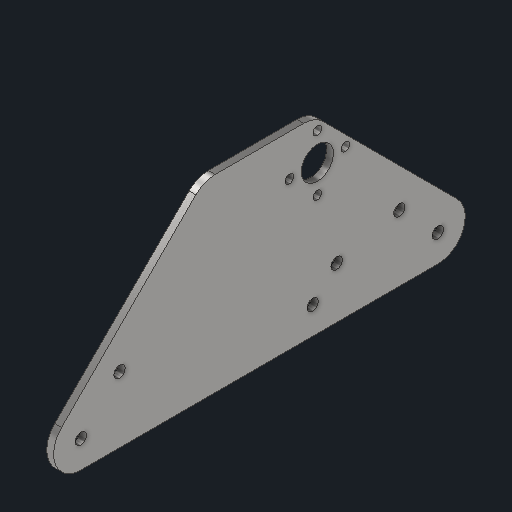
# Autodesk Inventor part: HipPivotPlate
Saved by Autodesk Inventor 2026.1 (Build 301233020, 233B)
## iProperties
Created: 2023-04-06
Part Number: HipPivotPlate
Material: Aluminum 6061
Document SubType Name: Modeling
Designer: Dave
Density: 2.7 g/cm^3
Appearance: Galvanized
Mass: 96.5969 g
Surface Area: 244.776 cm^2
Volume: 35.7766 cm^3
Author: Dave
Autodesk Inventor part; units mm, degrees
ref_plane "YZ Plane" through (0, 0, 0) normal (1, 0, 0) x (0, 1, 0)
ref_plane "XZ Plane" through (0, 0, 0) normal (0, 1, 0) x (-1, 0, 0)
ref_plane "XY Plane" through (0, 0, 0) normal (0, 0, 1) x (1, 0, 0)
sketch "Sketch1" plane through (0, 0, 0) normal (1, 0, 0) x (0, 1, 0)
  circle A0 centre (0, 0) radius 7.5075
  circle A1 centre (-56.0605, -56.0605) radius 2.65
  circle A2 centre (-38.1, -38.1) radius 2.65
  circle A3 centre (-47.0803, 100.9618) radius 2.65
  circle A4 centre (-56.0605, 109.942) radius 2.65
  circle A5 centre (-38.1, 91.9815) radius 2.65
  circle A6 centre (-47.0803, -47.0803) radius 2.65
  line L0 (-47.0803, 100.9618) -> (6.8013, 47.0803) construction
  line L1 (-35.921, 35.921) -> (0, 0) construction
  line L2 (0, 0) -> (-35.921, -35.921) construction
  line L3 (0, 0) -> (12.7, 0) construction
  line L4 (-47.0803, 118.9223) -> (15.3303, 56.5118)
  line L5 (19.05, 47.5315) -> (19.05, 6.35)
  line L6 (-68.7605, -56.0605) -> (-68.7605, 109.942)
  arc A7 (19.05, 47.5315) -> (15.3303, 56.5118) centre (6.35, 47.5315) ccw
  arc A8 (-47.0803, 118.9223) -> (-68.7605, 109.942) centre (-56.0605, 109.942) ccw
  line L7 (-47.0803, -65.0408) -> (15.3303, -2.6303)
  arc A9 (15.3303, -2.6303) -> (19.05, 6.35) centre (6.35, 6.35) ccw
  arc A10 (-68.7605, -56.0605) -> (-47.0803, -65.0408) centre (-56.0605, -56.0605) ccw
  line L8 (-26.9408, -8.9802) -> (-44.9013, -26.9407) projected
  line L9 (-44.9013, -26.9407) -> (-284.0015, 212.1595) projected
  line L10 (-266.041, 230.12) -> (-284.0015, 212.1595) projected
  line L11 (-26.9408, -8.9802) -> (-266.041, 230.12) projected
  circle A11 centre (-56.0605, 2.179) radius 2.65
  circle A12 centre (-44.9013, -8.9802) radius 2.65
  line L12 (-56.0605, 2.179) -> (-44.9013, -8.9802) construction
  point P0 (19.05, 1.0895)
  point P1 (-68.7605, -86.721)
  point P2 (-68.7605, 32.8395)
  dimension "d0" = 15.015
  dimension "d1" = 5.3
  dimension "d2" = 5.3
  dimension "d3" = 5.3
  dimension "d4" = 5.3
  dimension "d5" = 5.3
  dimension "d6" = 5.3
  dimension "d8" = 38.1
  dimension "d10" = 38.1
  dimension "d11" = 12.7
  dimension "d12" = 12.7
  dimension "d13" = 38.1
  dimension "d14" = 12.7
  dimension "d15" = 12.7
  dimension "d16" = 12.7
  dimension "d18" = 19.05
  dimension "d19" = 45
  dimension "d20" = 12.7
  dimension "d21" = 12.7
  dimension "d24" = 12.7
  dimension "d25" = 12.7
  dimension "d27" = 12.7
  dimension "d29" = 12.7
  dimension "d34" = 12.7
  dimension "d47" = 12.7
  dimension "d49" = 50.8
  dimension "d50" = 76.2
  dimension "d51" = 12.7
  constraints: 18 end point, 13 centre point, 9 point on line, 8 point on circle, 8 tangent, 4 parallel, 3 equal radius, 3 perpendicular, 1 coincident, 1 horizontal, 1 vertical
  measures "d0" diameter of A0
  measures "d1" diameter of A1
  measures "d2" diameter of A2
  measures "d3" diameter of A3
  measures "d4" diameter of A4
  measures "d5" diameter of A5
  measures "d6" diameter of A6
  measures "d8" distance between parallel lines of L1 L0
  measures "d10" horizontal distance of A5.centre point (0, 0)
  measures "d11" distance of A5.centre L0.start
  measures "d12" distance of L0.start A4.centre
  measures "d13" horizontal distance of A2.centre point (0, 0)
  measures "d14" distance of A6.centre A2.centre
  measures "d15" distance of A1.centre A6.centre
  measures "d16" distance from line of L4 A5.centre
  measures "d18" distance from line of L5 point (0, 0)
  measures "d19" angle of L5 L4
  measures "d20" distance from line of L6 A4.centre
  measures "d21" radius of A7
  measures "d24" radius of A9
  measures "d25" distance from line of L7 A1.centre
  measures "d27" distance between parallel lines of L11 L12
  measures "d29" distance from line of L8 L12.end
  measures "d34" distance from line of L6 L12.start
  measures "d47" radius of A8
  measures "d49" distance of L1.start L1.end
  measures "d50" distance of L0.start L0.end
  measures "d51" distance of L1.end L3.end
extrude "Extrusion2" add sketch "Sketch1" along normal blind 3.175 contours A3 | A6 | L4 A7 L5 A9 L7 A10 L6 L9 L8 L11 A8 | L11 L8 L9 L6
sketch "Sketch3" plane through (3.175, 0, 0) normal (1, 0, 0) x (0, 0, -1)
  circle A0 centre (0, 0) radius 7.5075 projected
  circle A1 centre (0, 0) radius 13 construction
  circle A2 centre (-0.0008, 13) radius 2
  line L0 (-6.35, 19.05) -> (-47.5315, 19.05) projected
  circle A3 centre (-13, -0.0008) radius 2
  circle A4 centre (0.0008, -13) radius 2
  circle A5 centre (13, 0.0008) radius 2
  dimension "d37" = 26
  dimension "d38" = 4
  dimension "d42" = 360
  constraints: 4 centre point, 3 coincident, 14 other
  measures "d38" diameter of A2
extrude "Extrusion3" cut sketch "Sketch3" against normal blind 25.4 contours A2 | A3 | A4 | A5
equation "\"d12\" = d11"
equation "\"d13\" = d10"
equation "\"d14\" = d11"
equation "\"d15\" = d11"
body "Solid2"
